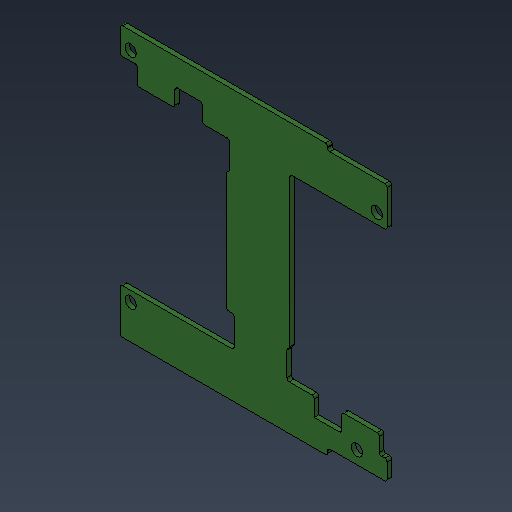
# Autodesk Inventor part: PCB_InterfaceBoard
Saved by Autodesk Inventor 2026.2 (Build 302298010, 298A)
## iProperties
Created: 2026-04-14
Part Number: PCB_InterfaceBoard
Material: Generic
Document SubType Name: Modeling
Designer: szymo
Density: 1 g/cm^3
Appearance: Default(1)
Author: szymo
Autodesk Inventor part; units mm, degrees
ref_plane "YZ Plane" through (0, 0, 0) normal (1, 0, 0) x (0, 1, 0)
ref_plane "XZ Plane" through (0, 0, 0) normal (0, 1, 0) x (-1, 0, 0)
ref_plane "XY Plane" through (0, 0, 0) normal (0, 0, 1) x (1, 0, 0)
sketch "Sketch1" plane through (0, 0, 0) normal (0, 0, 1) x (1, 0, 0)
  line L0 (13.7023, 4) -> (22.3525, 4)
  line L1 (22.3525, 0) -> (59.3371, 0)
  line L2 (59.3371, 0) -> (59.3371, 9.3)
  line L3 (59.3371, 9.3) -> (0, 9.3)
  line L4 (0, 4) -> (0, 9.3)
  line L5 (2.4551, 0) -> (13.7023, 0)
  line L6 (0, -38.4) -> (39.318, -38.4)
  line L7 (0, -38.4) -> (0, -47.7)
  line L8 (0, -47.7) -> (59.3371, -47.7)
  line L9 (59.3371, -42.4) -> (59.3371, -47.7)
  line L10 (59.3371, -42.4) -> (58.882, -42.4)
  line L11 (58.882, -42.4) -> (58.882, -38.4)
  line L12 (47.6348, -38.4) -> (58.882, -38.4)
  line L13 (47.6348, -42.4) -> (39.318, -42.4)
  line L14 (39.0735, -33.15) -> (39.0735, -5.25)
  line L15 (39.0735, -5.25) -> (39.9371, -5.25)
  line L16 (39.9371, -5.25) -> (39.9371, -33.15)
  line L17 (39.9371, -33.15) -> (39.0735, -33.15)
  line L18 (22.2636, -5.25) -> (22.2636, -33.15)
  line L19 (22.2636, -33.15) -> (21.4, -33.15)
  line L20 (21.4, -33.15) -> (21.4, -5.25)
  line L21 (21.4, -5.25) -> (22.2636, -5.25)
  line L22 (21.4, 0) -> (21.4, -38.4)
  line L23 (39.9371, -38.4) -> (39.9371, 0)
  line L24 (39.9371, 0) -> (62.3371, 0)
  line L25 (58.8371, 9.1) -> (58.8371, 0.5)
  line L26 (58.8371, 0.5) -> (37.5735, 0.5)
  line L27 (37.5735, 0.5) -> (37.5735, -6.25)
  line L28 (37.5735, -6.25) -> (37.5735, -6.25)
  line L29 (37.5735, -6.25) -> (37.5735, -32.65)
  line L30 (36.9371, -32.65) -> (36.9371, -38.9)
  line L31 (58.8371, -42.9) -> (58.8371, -47.2)
  line L32 (58.8371, -47.2) -> (45.8371, -47.2)
  line L33 (0.5, -48.7) -> (0.5, -38.9)
  line L34 (0.5, -38.9) -> (25.4, -38.9)
  line L35 (25.4, -38.9) -> (25.4, -32.15)
  line L36 (25.4, -32.15) -> (23.7636, -32.15)
  line L37 (23.7636, -32.15) -> (23.7636, -5.75)
  line L38 (23.7636, -5.75) -> (24.4, -5.75)
  line L39 (24.4, -5.75) -> (24.4, 0.5)
  line L40 (0.5, 4.5) -> (0.5, 9.1)
  line L41 (37.5735, -32.65) -> (36.9371, -32.65)
  circle A0 centre (2.75, -41.15) radius 1.75
  circle A1 centre (52.2136, -44.4) radius 1.75
  circle A2 centre (56.5871, 2.75) radius 1.75
  circle A3 centre (2.75, 6.55) radius 1.75
  circle A4 centre (56.5871, 2.75) radius 1.25
  circle A5 centre (52.2136, -44.4) radius 1.25
  circle A6 centre (2.75, -41.15) radius 1.25
  circle A7 centre (2.75, 6.55) radius 1.25
  line L42 (12.4424, 4.5) -> (12.4424, 0.5)
  line L43 (12.4424, 0.5) -> (4.212, 0.5)
  line L44 (4.212, 0.5) -> (4.212, 4.5)
  line L45 (4.212, 4.5) -> (0.5, 4.5)
  line L46 (58.8371, -42.9) -> (57.125, -42.9)
  line L47 (57.125, -42.9) -> (57.125, -38.9)
  line L48 (57.125, -38.9) -> (48.8947, -38.9)
  line L49 (48.8947, -38.9) -> (48.8947, -42.9)
  line L50 (39.318, -42.4) -> (39.318, -38.4)
  line L51 (47.6348, -38.4) -> (47.6348, -42.4)
  line L52 (22.3525, 4) -> (22.3525, 0)
  spline S0 degree 2 poles (41.0471, 11.3) (40.5342, 11.2191) (40.0213, 11.3) knots 0 0 0 1 1 1 weights 1 1.01269 1
  line L53 (0, 11.3) -> (40.0213, 11.3)
  line L54 (0, 9.3) -> (0, 11.3)
  line L55 (0, 9.3) -> (46.3371, 9.3)
  line L56 (46.3371, 9.3) -> (46.3371, 11.3)
  line L57 (41.0471, 11.3) -> (46.3371, 11.3)
  spline S1 degree 2 poles (20.1962, -49.7) (20.5821, -49.6542) (20.9681, -49.7) knots 0 0 0 1 1 1 weights 1 1.007125 1
  line L58 (46.3371, -49.7) -> (20.9681, -49.7)
  line L59 (46.3371, -47.7) -> (46.3371, -49.7)
  line L60 (0, -47.7) -> (46.3371, -47.7)
  line L61 (0, -47.7) -> (0, -49.7)
  line L62 (20.1962, -49.7) -> (0, -49.7)
  line L63 (45.8371, -48.7) -> (0.5, -48.7)
  line L64 (45.8371, -47.2) -> (45.8371, -48.7)
  line L65 (45.8371, 9.1) -> (58.8371, 9.1)
  line L66 (45.8371, 9.1) -> (45.8371, 10.3)
  line L67 (45.8371, 10.3) -> (0.5, 10.3)
  line L68 (0.5, 10.3) -> (0.5, 9.1)
  line L69 (3.712, 4) -> (3.712, 0)
  line L70 (12.9424, 0) -> (12.9424, 4)
  line L71 (17.9365, 4) -> (17.9365, 0)
  line L72 (12.4424, 4.5) -> (18.4365, 4.5)
  line L73 (18.4365, 4.5) -> (18.4365, 0.5)
  line L74 (18.4365, 0.5) -> (24.4, 0.5)
  line L75 (43.4006, -42.4) -> (43.4006, -38.4)
  line L76 (48.3947, -38.4) -> (48.3947, -42.4)
  line L77 (57.625, -42.4) -> (57.625, -38.4)
  line L78 (36.9371, -38.9) -> (42.9006, -38.9)
  line L79 (42.9006, -38.9) -> (42.9006, -42.9)
  line L80 (42.9006, -42.9) -> (48.8947, -42.9)
  point P0 (0, 0)
  point P1 (37.5735, 0)
  point P2 (36.9371, -38.4)
  dimension "d1" = 0.5
  dimension "d3" = 0.5
  dimension "d5" = 0.5
  dimension "d7" = 0.5
  dimension "d8" = 0.5
  dimension "d10" = 0.5
  dimension "d11" = 0.5
  dimension "d16" = 1.5
  dimension "d17" = 1.5
  dimension "d18" = 3
  dimension "d19" = 0.5
  dimension "d20" = 1
  dimension "d21" = 1
  dimension "d22" = 0.5
  dimension "d23" = 2.3636
  dimension "d24" = 3
  dimension "d25" = 4
  dimension "d29" = 2.5
  dimension "d30" = 2.5
  dimension "d31" = 2.5
  dimension "d32" = 2.5
  dimension "d35" = 0.5
  dimension "d40" = 0.5
  dimension "d42" = 0.5
  dimension "d44" = 0.5
  dimension "d45" = 1
  dimension "d47" = 0.2
  dimension "d48" = 0.5
  dimension "d49" = 1
  dimension "d50" = 0
  dimension "d51" = 0.5
  dimension "d52" = 0.5
  dimension "d53" = 0.5
  dimension "d54" = 0.5
  dimension "d55" = 0.5
  dimension "d56" = 0.5
  dimension "d57" = 0.5
  dimension "d59" = 0.5
  dimension "d60" = 0.5
  dimension "d61" = 0.5
  dimension "d62" = 0.5
  constraints: 109 end point, 19 perpendicular, 18 vertical, 10 horizontal, 4 centre point, 4 coincident, 3 parallel, 26 other
  measures "d1" distance between parallel lines of L26 L24
  measures "d3" distance between parallel lines of L2 L25
  measures "d5" distance between parallel lines of L4 L40
  measures "d7" distance between parallel lines of L6 L34
  measures "d8" distance between parallel lines of L7 L33
  measures "d10" distance between parallel lines of L9 L31
  measures "d11" distance between parallel lines of L8 L32
  measures "d16" distance between parallel lines of L37 L18
  measures "d17" distance between parallel lines of L14 L29
  measures "d18" distance between parallel lines of L39 L22
  measures "d19" distance between parallel lines of L38 L21
  measures "d20" distance between parallel lines of L28 L15
  measures "d21" distance between parallel lines of L36 L19
  measures "d22" distance between parallel lines of L17 L41
  measures "d23" distance between parallel lines of L27 L23
  measures "d24" distance between parallel lines of L30 L23
  measures "d25" distance between parallel lines of L22 L35
  measures "d29" diameter of A4
  measures "d30" diameter of A5
  measures "d31" diameter of A6
  measures "d32" diameter of A7
  measures "d35" distance between parallel lines of L5 L43
  measures "d40" distance between parallel lines of L12 L48
  measures "d42" distance between parallel lines of L10 L46
  measures "d44" distance between parallel lines of L59 L64
  measures "d45" distance between parallel lines of L62 L63
  measures "d47" distance between parallel lines of L3 L65
  measures "d48" distance between parallel lines of L56 L66
  measures "d49" distance between parallel lines of L53 L67
  measures "d50" distance between parallel lines of L29 L27
  measures "d51" distance between parallel lines of L44 L69
  measures "d52" distance from line of L45 L69.start
  measures "d53" distance between parallel lines of L42 L70
  measures "d54" distance between parallel lines of L1 L74
  measures "d55" distance between parallel lines of L71 L73
  measures "d56" distance between parallel lines of L72 L0
  measures "d57" distance between parallel lines of L76 L49
  measures "d59" distance between parallel lines of L78 L6
  measures "d60" distance between parallel lines of L75 L79
  measures "d61" distance between parallel lines of L13 L80
  measures "d62" distance between parallel lines of L77 L47
extrude "Extrusion1" add sketch "Sketch1" along normal blind 1 contours L73 L72 L42 L43 L44 L45 L40 L68 L3 L66 L65 L25 L26 L27 L1 L39 L74 L52 L0 | L0 L52 L74 L73 | L1 L27 L29 L41 L30 L6 L35 L36 L37 L38 L39 | L68 L67 L66 L3 | L30 L78 L50 L13 L79 L80 L49 L48 L47 L46 L31 L32 L64 L8 L33 L34 L35 L6 | L78 L79 L13 L50 | L8 L64 L63 L33 | A0 | A1 | A2 | A3
fillet "Fillet1" radius 0.5 33 edges at (58.8371, -47.2, 0.5) (58.8371, -42.9, 0.5) (0.5, -38.9, 0.5) (25.4, -38.9, 0.5) (25.4, -32.15, 0.5) (23.7636, -32.15, 0.5) (23.7636, -5.75, 0.5) (24.4, -5.75, 0.5) (24.4, 0.5, 0.5) (0.5, 4.5, 0.5) (58.8371, 9.1, 0.5) (58.8371, 0.5, 0.5) (37.5735, 0.5, 0.5) (37.5735, -32.65, 0.5) (36.9371, -32.65, 0.5) (36.9371, -38.9, 0.5) (4.212, 4.5, 0.5) (4.212, 0.5, 0.5) (12.4424, 4.5, 0.5) (12.4424, 0.5, 0.5) (48.8947, -42.9, 0.5) (48.8947, -38.9, 0.5) (57.125, -38.9, 0.5) (57.125, -42.9, 0.5) (45.8371, -47.2, 0.5) (45.8371, -48.7, 0.5) (0.5, -48.7, 0.5) (45.8371, 9.1, 0.5) (45.8371, 10.3, 0.5) (0.5, 10.3, 0.5) (42.9006, -38.9, 0.5) (18.4365, 4.5, 0.5) (18.4365, 0.5, 0.5)
equation "\"d5\" = d1"
equation "\"d7\" = d1"
equation "\"d8\" = d1"
equation "\"d10\" = d1"
equation "\"d30\" = d29"
equation "\"d31\" = d29"
equation "\"d32\" = d29"
equation "\"d40\" = d1"
body "Solid1"
